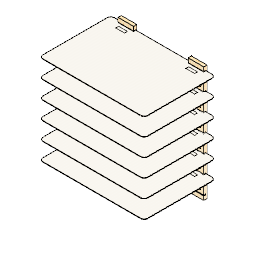
MKFG_ModularCoolingRacks v8 (Autodesk Fusion 360 design; units mm, degrees)
Autodesk Fusion 360 part; units mm, degrees
note: some values were not read from the file. Chosen so that the rebuilt part matches the saved one: which bodies a step acts on.
sketch "Sketch1" plane through (0, 0, 0) normal (0, 0, 1) x (1, 0, 0)
  line L0 (-44.45, 330.2) -> (44.45, 330.2)
  line L1 (44.45, 330.2) -> (44.45, -330.2)
  line L2 (44.45, -330.2) -> (-44.45, -330.2)
  line L3 (-44.45, -330.2) -> (-44.45, 330.2)
  line L4 (-44.45, 306.3875) -> (44.45, 306.3875)
  line L5 (-44.45, 303.2125) -> (44.45, 303.2125)
  line L6 (-44.45, -306.3875) -> (44.45, -306.3875)
  line L7 (-44.45, -303.2125) -> (44.45, -303.2125)
  line L8 (-44.45, 0) -> (44.45, 0) construction
  line L9 (-44.45, -3.175) -> (44.45, -3.175)
  line L10 (-44.45, 3.175) -> (44.45, 3.175)
  line L11 (-44.45, -200.025) -> (44.45, -200.025)
  line L12 (-44.45, -206.375) -> (44.45, -206.375)
  line L13 (-44.45, -98.425) -> (44.45, -98.425)
  line L14 (-44.45, -104.775) -> (44.45, -104.775)
  line L15 (-44.45, 104.775) -> (44.45, 104.775)
  line L16 (-44.45, 98.425) -> (44.45, 98.425)
  line L17 (-44.45, 206.375) -> (44.45, 206.375)
  line L18 (-44.45, 200.025) -> (44.45, 200.025)
  line L19 (0, 303.2125) -> (0, 206.375) construction
  circle A0 centre (0, 254.7938) radius 3.175
  line L20 (0, -206.375) -> (0, -303.2125) construction
  circle A1 centre (0, -254.7938) radius 3.175
  dimension "d1" = 88.9
  dimension "d2" = 660.4
  dimension "d3" = 44.45
  dimension "d4" = 330.2
  dimension "d5" = 23.8125
  dimension "d6" = 3.175
  dimension "d7" = 23.8125
  dimension "d8" = -3.175
  dimension "d9" = 3.175
  dimension "d10" = -3.175
  dimension "d13" = 0
  dimension "d14" = 101.6
  dimension "d20" = 6.35
  dimension "d21" = 6.35
  constraint horizontal L0
  constraint vertical L1
  constraint horizontal L2
  constraint vertical L3
  constraint coincident L3 L4.start
  constraint coincident L1 L4.end
  constraint perpendicular L1 L4
  constraint coincident L3 L6.start
  constraint coincident L1 L6.end
  constraint perpendicular L1 L6
  constraint midpoint L3 L8.start
  constraint midpoint L1 L8.end
  constraint midpoint L5 L19.start
  constraint midpoint L17 L19.end
  constraint perpendicular L17 L19
  constraint coincident L19 A0.centre
  constraint midpoint L12 L20.start
  constraint midpoint L7 L20.end
  constraint perpendicular L7 L20
  constraint midpoint L20 A1.centre
  constraint coincident L1 L12.end
  constraint coincident L3 L12.start
  constraint coincident L1 L7.end
  constraint coincident L1 L5.end
  constraint coincident L3 L5.start
  constraint coincident L1 L17.end
  constraint midpoint L19 A0.centre
  measures "d1" distance of L0.start L0.end
  measures "d2" distance of L0.start L2.end
  measures "d3" distance of origin L3
  measures "d4" distance of origin L0
  measures "d5" distance of L0 L4
  measures "d7" distance of L2 L6
  measures "d20" diameter of A0
  measures "d21" diameter of A1
extrude "Extrude1" add sketch "Sketch1" along normal blind 19.05 contours L0 L1 L3 L4 | L1 L3 L4 L5 | L1 L3 L5 L17 | L1 L3 L17 L18 | L1 L3 L15 L18 | L1 L3 L15 L16 | L1 L3 L10 L16 | L1 L3 L9 L10 | L1 L3 L9 L13 | L1 L3 L13 L14 | L1 L3 L11 L14 | L1 L3 L11 L12 | L1 L3 L7 L12 | L1 L3 L6 L7 | L1 L2 L3 L6 | A0 | A1 makes body 1
extrude "Extrude2" cut sketch "Sketch1" against normal blind 12.7 from surface at 19.05 contours L1 L3 L4 L5 | L1 L3 L17 L18 | L1 L3 L15 L16 | L1 L3 L9 L10 | L1 L3 L13 L14 | L1 L3 L11 L12 | L1 L3 L6 L7 bodies 1
extrude "Extrude3" cut sketch "Sketch1" along normal up to surface (19.05 mm away) contours A0 | A1 bodies 1
sketch "Sketch2" plane through (-44.45, 0, 0) normal (-1, 0, 0) x (0, 0, 1)
  line L0 (6.35, -98.425) -> (19.05, -98.425)
  line L1 (19.05, -98.425) -> (19.05, -3.175)
  line L2 (19.05, -3.175) -> (6.35, -3.175)
  line L3 (6.35, -3.175) -> (6.35, 3.175)
  line L4 (6.35, 3.175) -> (19.05, 3.175)
  line L5 (19.05, 3.175) -> (19.05, 98.425)
  line L6 (19.05, 98.425) -> (6.35, 98.425)
  line L7 (6.35, 98.425) -> (6.35, 104.775)
  line L8 (6.35, 104.775) -> (19.05, 104.775)
  line L9 (19.05, 104.775) -> (19.05, 200.025)
  line L10 (19.05, 200.025) -> (6.35, 200.025)
  line L11 (6.35, 200.025) -> (6.35, 206.375)
  line L12 (6.35, 206.375) -> (19.05, 206.375)
  line L13 (19.05, 206.375) -> (19.05, 303.2125)
  line L14 (19.05, 303.2125) -> (6.35, 303.2125)
  line L15 (6.35, 303.2125) -> (6.35, 306.3875)
  line L16 (6.35, 306.3875) -> (19.05, 306.3875)
  line L17 (19.05, 306.3875) -> (19.05, 330.2)
  line L18 (19.05, 330.2) -> (0, 330.2)
  line L19 (0, 330.2) -> (0, -330.2)
  line L20 (0, -330.2) -> (19.05, -330.2)
  line L21 (19.05, -330.2) -> (19.05, -306.3875)
  line L22 (19.05, -306.3875) -> (6.35, -306.3875)
  line L23 (6.35, -306.3875) -> (6.35, -303.2125)
  line L24 (6.35, -303.2125) -> (19.05, -303.2125)
  line L25 (19.05, -303.2125) -> (19.05, -206.375)
  line L26 (19.05, -206.375) -> (6.35, -206.375)
  line L27 (6.35, -206.375) -> (6.35, -200.025)
  line L28 (6.35, -200.025) -> (19.05, -200.025)
  line L29 (19.05, -200.025) -> (19.05, -104.775)
  line L30 (19.05, -104.775) -> (6.35, -104.775)
  line L31 (6.35, -104.775) -> (6.35, -98.425)
  line L32 (19.05, 196.025) -> (31.75, 196.025)
  line L33 (31.75, 196.025) -> (31.75, 202.375)
  line L34 (31.75, 202.375) -> (57.15, 202.375)
  line L35 (57.15, 202.375) -> (19.05, 121.025)
  dimension "d24" = 12.7
  dimension "d25" = 6.35
  dimension "d26" = 25.4
  dimension "d27" = 75
  dimension "d28" = 4
  constraint coincident L9 L32.start
  constraint perpendicular L9 L32
  constraint perpendicular L32 L33
  constraint perpendicular L33 L34
  constraint coincident L9 L35.end
  measures "d24" distance of L32.start L32.end
  measures "d25" distance of L32.end L33.end
  measures "d26" distance of L33.end L34.end
  measures "d27" distance of L32.start L35.end
  measures "d28" distance of L10 L32
extrude "Extrude4" add sketch "Sketch2" against normal blind 50.8 from surface at -19.05 separate body contours L9 L32 L33 L34 L35 makes body 2
fillet "Fillet1" radius 3.5 3 edges at (0, 202.375, 31.75) (0, 196.025, 31.75) (0, 202.375, 57.15) on bodies 2
chamfer "Chamfer2" distance 0.5 distance2 0.5 2 edges at (0, 121.025, 19.05) (0, 196.025, 19.05) 2 faces at (-25.4, 171.5539, 34.4568) (25.4, 171.5539, 34.4568) measured on face at (-8.4667, 171.9354, 42.8937) measured on face at (8.4667, 146.025, 19.05) on bodies 2
sketch "Sketch3" plane through (0, 0, 19.05) normal (0, 0, -1) x (-1, 0, 0)
  line L0 (24.9, 195.525) -> (-24.9, 195.525)
  line L1 (-24.9, 195.525) -> (-24.9, 121.525)
  line L2 (-24.9, 121.525) -> (24.9, 121.525)
  line L3 (24.9, 121.525) -> (24.9, 195.525)
  line L4 (0, 195.525) -> (0, 121.525) construction
  line L5 (-1.9, 187.375) -> (-1.9, 180.375)
  arc A0 (-1.9, 180.375) -> (1.9, 180.375) centre (0, 180.375) ccw
  line L6 (1.9, 180.375) -> (1.9, 187.375)
  arc A1 (1.9, 187.375) -> (-1.9, 187.375) centre (0, 187.375) ccw
  line L7 (0, 187.375) -> (0, 180.375) construction
  line L8 (-1.9, 142.375) -> (-1.9, 135.375)
  arc A2 (-1.9, 135.375) -> (1.9, 135.375) centre (0, 135.375) ccw
  line L9 (1.9, 135.375) -> (1.9, 142.375)
  arc A3 (1.9, 142.375) -> (-1.9, 142.375) centre (0, 142.375) ccw
  line L10 (0, 142.375) -> (0, 135.375) construction
  line L11 (24.9, 202.375) -> (-24.9, 202.375)
  line L12 (-5.9, 187.375) -> (-5.9, 180.375)
  arc A4 (-5.9, 180.375) -> (5.9, 180.375) centre (0, 180.375) ccw
  line L13 (5.9, 180.375) -> (5.9, 187.375)
  arc A5 (5.9, 187.375) -> (-5.9, 187.375) centre (0, 187.375) ccw
  line L14 (-5.9, 142.375) -> (-5.9, 135.375)
  arc A6 (-5.9, 135.375) -> (5.9, 135.375) centre (0, 135.375) ccw
  line L15 (5.9, 135.375) -> (5.9, 142.375)
  arc A7 (5.9, 142.375) -> (-5.9, 142.375) centre (0, 142.375) ccw
  dimension "d42" = 3.8
  dimension "d43" = 3.8
  dimension "d44" = 45
  dimension "d45" = 7
  dimension "d46" = 7
  dimension "d47" = 15
  dimension "d48" = 4
  dimension "d49" = 4
  constraint midpoint L0 L4.start
  constraint midpoint L2 L4.end
  constraint tangent L5 A0
  constraint tangent A0 L6
  constraint parallel L5 L6
  constraint tangent L6 A1
  constraint tangent L5 A1
  constraint perpendicular L0 L7
  constraint coincident L4 A1.centre
  constraint tangent L8 A2
  constraint tangent A2 L9
  constraint parallel L8 L9
  constraint tangent L9 A3
  constraint tangent L8 A3
  constraint parallel L4 L10
  constraint coincident L4 A3.centre
  measures "d42" diameter of A0
  measures "d43" diameter of A2
  measures "d44" distance of A1.centre A3.centre
  measures "d45" distance of L5.start L5.end
  measures "d46" distance of L8.start L8.end
  measures "d47" distance of A1.centre L11
extrude "Extrude5" cut sketch "Sketch3" against normal blind 40 contours L5 A0 L6 A1 | L8 A2 L9 A3 bodies 2
extrude "Extrude6" cut sketch "Sketch3" against normal blind 40 from surface at -3.175 contours L12 A4 L13 A5 | L14 A6 L15 A7 bodies 2
sketch "Sketch4" plane through (0, 0, 19.05) normal (0, 0, 1) x (1, 0, 0)
  line L0 (44.45, 200.025) -> (-44.45, 200.025)
  line L1 (-44.45, 200.025) -> (-44.45, 104.775)
  line L2 (-44.45, 104.775) -> (44.45, 104.775)
  line L3 (44.45, 104.775) -> (44.45, 200.025)
  line L4 (44.45, 201.625) -> (-44.45, 201.625)
  line L5 (0, 200.025) -> (0, 185.025) construction
  line L6 (0, 185.025) -> (0, 140.025) construction
  circle A0 centre (0, 185.025) radius 1.5875
  circle A1 centre (0, 140.025) radius 1.5875
  line L7 (5, 140.025) -> (5, 201.625)
  arc A2 (5, 201.625) -> (-5, 201.625) centre (0, 201.625) ccw
  line L8 (-5, 201.625) -> (-5, 140.025)
  arc A3 (-5, 140.025) -> (5, 140.025) centre (0, 140.025) ccw
  line L9 (0, 140.025) -> (0, 201.625) construction
  line L10 (44.45, 201.625) -> (44.45, 200.025)
  line L11 (-44.45, 201.625) -> (-44.45, 200.025)
  line L12 (44.45, 201.625) -> (46.05, 201.625)
  line L13 (46.05, 201.625) -> (46.05, 196.625)
  line L14 (-44.45, 201.625) -> (-46.05, 201.625)
  line L15 (-46.05, 201.625) -> (-46.05, 196.625)
  line L16 (-46.05, 196.625) -> (-5, 170.825)
  line L17 (46.05, 196.625) -> (5, 170.825)
  dimension "d55" = 1.6
  dimension "d56" = 15
  dimension "d57" = 45
  dimension "d58" = 3.175
  dimension "d59" = 3.175
  dimension "d60" = 10
  dimension "d61" = 1.6
  dimension "d62" = 5
  dimension "d63" = 1.6
  dimension "d64" = 5
  constraint midpoint L0 L5.start
  constraint perpendicular L0 L5
  constraint parallel L5 L6
  constraint coincident L5.end L6.start
  constraint coincident L6.end A1.centre
  constraint tangent L7 A2
  constraint tangent A2 L8
  constraint parallel L7 L8
  constraint tangent L8 A3
  constraint tangent L7 A3
  constraint midpoint L4 A2.centre
  constraint perpendicular L4 L9
  constraint coincident L0.start L3.end
  constraint coincident L0.end L1.start
  constraint perpendicular L0 L10
  constraint perpendicular L10 L12
  constraint perpendicular L12 L13
  constraint perpendicular L11 L14
  constraint perpendicular L14 L15
  constraint midpoint L8 L16.end
  constraint midpoint L7 L17.end
  measures "d56" distance of L5.start L5.end
  measures "d57" distance of L5.end L6.end
  measures "d58" diameter of A0
  measures "d59" diameter of A1
  measures "d60" diameter of A2
  measures "d61" distance of L4.start L12.end
  measures "d62" distance of L12.end L13.end
  measures "d63" distance of L4.end L14.end
  measures "d64" distance of L14.end L15.end
extrude "Extrude7" add sketch "Sketch4" along normal blind 1 separate body contours L0 L3 L7 L17 | L3 L10 L12 L13 L17 | L0 L4 L7 L10 | L0 L7 L8 A3 | L0 L4 L7 L8 | L0 L1 L8 L16 | L0 L4 L8 L11 | L1 L11 L14 L15 L16 makes body 3
extrude "Extrude8" add sketch "Sketch4" against normal blind 5 contours L3 L10 L12 L13 L17 | L0 L4 L7 L10 | L0 L4 L7 L8 | L0 L4 L8 L11 | L1 L11 L14 L15 L16 bodies 3
fillet "Fillet4" radius 0.8 2 edges at (-44.45, 195.6194, 16.55) (44.45, 195.6194, 16.55) on bodies 3
copy_body "CopyPasteBodies1" bodies 1 2 makes body 4 makes body 5
move_body "Move1" bodies 4 5 to x (1, 0, 0) y (0, 1, 0) z (0, 0, 1) at (400, 0, 0)
pattern_linear "R-Pattern1" count 5 spacing 101.6 along (0, -1, 0) of bodies 2 5 makes body 6 at (18.417, 52.9004, 34.7281) makes body 7 at (18.417, -48.6996, 34.7281) makes body 8 at (18.417, -150.2996, 34.7281) makes body 9 at (18.417, -251.8996, 34.7281) makes body 10 at (418.417, 52.9004, 34.7281) makes body 11 at (418.417, -48.6996, 34.7281) makes body 12 at (418.417, -150.2996, 34.7281) makes body 13 at (418.417, -251.8996, 34.7281)
sketch "Sketch5" plane through (0, 200.025, 0) normal (0, 1, 0) x (-1, 0, 0)
  line L0 (44.45, 19.05) -> (-44.45, 19.05)
  line L1 (-44.45, 19.05) -> (-44.45, 6.35)
  line L2 (-44.45, 6.35) -> (44.45, 6.35)
  line L3 (44.45, 6.35) -> (44.45, 19.05)
  line L4 (-355.55, 19.05) -> (-444.45, 19.05)
  line L5 (-444.45, 19.05) -> (-444.45, 6.35)
  line L6 (-444.45, 6.35) -> (-355.55, 6.35)
  line L7 (-355.55, 6.35) -> (-355.55, 19.05)
  line L8 (98.45, 6.35) -> (-498.45, 6.35)
  line L9 (-498.45, 6.35) -> (-498.45, 412.75)
  line L10 (-498.45, 412.75) -> (98.45, 412.75)
  line L11 (98.45, 412.75) -> (98.45, 6.35)
  line L12 (-355.55, 6.35) -> (-44.45, 6.35) construction
  point P0 (-200, 6.35)
  point P1 (-200, 6.35)
  dimension "d75" = 596.9
  dimension "d76" = 406.4
  constraint horizontal L8
  constraint vertical L9
  constraint horizontal L10
  constraint vertical L11
  constraint coincident L6.end L7.start
  constraint coincident L1.end L2.start
  constraint midpoint L12 P1
  constraint midpoint L8 P1
  constraint coincident P1 P0
  measures "d75" distance of L8.start L8.end
  measures "d76" distance of L8.start L10.end
extrude "Extrude9" add sketch "Sketch5" along normal blind 3.175 separate body makes body 14
fillet "Fillet5" radius 20 4 edges at (498.45, 201.6125, 412.75) (498.45, 201.6125, 6.35) (-98.45, 201.6125, 6.35) (-98.45, 201.6125, 412.75) on bodies 14
copy_body "CopyPasteBodies2" bodies 5 2 makes body 15 makes body 16
move_body "Move2" bodies 15 16 to x (1, 0, 0) y (0, 1, 0) z (0, 0, 1) at (0, 101.6, 0)
move_body "Move3" bodies 14 to x (1, 0, 0) y (0, 1, 0) z (0, 0, 1) at (0, 101.6, 0)
pattern_linear "R-Pattern2" count 6 spacing 101.6 along (0, -1, 0) of bodies 14 makes body 17 at (292.8167, 203.2, 277.2833) makes body 18 at (292.8167, 101.6, 277.2833) makes body 19 at (292.8167, 0, 277.2833) makes body 20 at (292.8167, -101.6, 277.2833) makes body 21 at (292.8167, -203.2, 277.2833)
move_body "Move4" bodies 14 17 18 19 21 20 to x (1, 0, 0) y (0, 1, 0) z (0, 0, 1) at (0, 1, 0)
hidden bodies 3
equation "d2 = 26\""
equation "d3 = d1 / 2"
equation "d4 = d2 / 2"
equation "d5 = 1\" - 1\" / 16"
equation "d6 = 1\" / 8"
equation "d7 = 1\" - 1\" / 16"
equation "d8 = -1\" / 8"
equation "d9 = 1\" / 8"
equation "d10 = -1\" / 8"
equation "d14 = 4\""
equation "d15 = 3\" / 4"
equation "d25 = 1\" / 4"
equation "d52 = -1\" / 8"
equation "d58 = 1\" / 8"
equation "d59 = 1\" / 8"
equation "d76 = 16\""
named bodies: "BWRack_1x4_WallPlate", "BWRackBraceA", "BWRackBraceDrillJig", "BWRack_1x4_WallPlate (1)", "BWRackBraceA (1)", "BWRackBraceA (2)", "BWRackBraceA (3)", "BWRackBraceA (4)", "BWRackBraceA (5)", "BWRackBraceA (1) (1)", "BWRackBraceA (1) (2)", "BWRackBraceA (1) (3)", "BWRackBraceA (1) (4)", "cooling_rack", "BWRackBraceA (1) (5)", "BWRackBraceA (2) (1)", "cooling_rack (1)", "cooling_rack (2)", "cooling_rack (3)", "cooling_rack (4)", "cooling_rack (5)"
